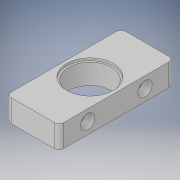
# Autodesk Inventor part: BearingBlock30mmRight
Saved by Autodesk Inventor 2018 (Build 220112000, 112)
## iProperties
Created: 2017-11-02
Part Number: BearingBlock30mmRight
Material: Generic
Document SubType Name: Modeling
Designer: snipe
Density: 1 g/cm^3
Appearance: Default
Author: snipe
Autodesk Inventor part; units mm, degrees
ref_plane "YZ Plane" through (0, 0, 0) normal (1, 0, 0) x (0, 1, 0)
ref_plane "XZ Plane" through (0, 0, 0) normal (0, 1, 0) x (-1, 0, 0)
ref_plane "XY Plane" through (0, 0, 0) normal (0, 0, 1) x (1, 0, 0)
sketch "Sketch1" plane through (0, 0, 0) normal (0, 1, 0) x (-1, 0, 0)
  line L0 (0, -53.34) -> (0, 53.34) projected
  line L1 (-24.5, 0) -> (24.5, 0) projected
  line L2 (24.5, 0) -> (-24.5, 0) projected
  line L3 (0, -53.34) -> (0, 53.34) projected
  line L4 (-17.5, 38.1) -> (-17.5, -38.1)
  line L5 (-17.5, -38.1) -> (17.5, -38.1)
  line L6 (17.5, -38.1) -> (17.5, 38.1)
  line L7 (17.5, 38.1) -> (-17.5, 38.1)
  line L8 (-17.5, -38.1) -> (17.5, 38.1) construction
  point P0 (0, 0)
  dimension "d1" = 76.2
  dimension "d2" = 35
  constraints: 10 end point, 2 parallel, 1 perpendicular, 1 vertical, 2 other
  measures "d1" distance of L4.start L4.end
  measures "d2" distance of L5.end L4.end
extrude "Extrusion1" add sketch "Sketch1" along normal mid plane 15
sketch "Sketch2" plane through (0, 7.5, 0) normal (0, 1, 0) x (1, 0, 0)
  point P0 (0, 0)
  point P1 (0, 0)
  constraints: 1 coincident
hole "Hole1" at (0, 7.5, 0) direction (0, -1, 0) diameter 28.575 end through all counterbore diameter 31.12 counterbore depth 1.588
fillet "Fillet1" radius 3.175 4 edges at (17.5, 0, 38.1) (17.5, 0, -38.1) (-17.5, 0, 38.1) (-17.5, 0, -38.1)
sketch "Sketch4" plane through (17.5, -7.5, -34.925) normal (1, 0, 0) x (0, 0, -1)
  line L0 (0, 15) -> (0, 0) projected
  line L1 (-69.85, 15) -> (0, 15) projected
  line L2 (-69.85, 0) -> (-69.85, 15) projected
  line L3 (0, 0) -> (-69.85, 0) projected
  line L4 (-69.85, 0) -> (0, 0)
  line L5 (0, 0) -> (0, 15)
  line L6 (0, 15) -> (-69.85, 15)
  line L7 (-69.85, 15) -> (-69.85, 0)
  line L8 (-50.485, 15) -> (-19.365, 15) projected
  line L9 (-34.925, 15) -> (-34.925, 0)
  line L10 (-69.85, 0) -> (-69.85, 15) projected
  line L11 (-69.85, 7.5) -> (0, 7.5)
  point P0 (-34.925, 7.5)
  point P1 (-53.975, 7.5)
  point P2 (-15.875, 7.5)
  dimension "d28" = 19.05
  dimension "d29" = 19.05
  constraints: 12 end point, 4 midpoint, 2 parallel, 2 point on line, 1 horizontal, 1 perpendicular
  measures "d28" distance from line of point (-53.975, 7.5) L9
  measures "d29" distance from line of L9 point (-15.875, 7.5)
hole "Hole3" at (17.5, 0, 19.05) at (17.5, 0, -19.05) direction (-1, 0, 0) diameter 6.35 end through all counterbore diameter 9.525 counterbore depth 6.35
body "Solid1"
